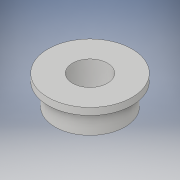
# Autodesk Inventor part: Roller Bearing
Saved by Autodesk Inventor 2019.4 (Build 234330000, 330)
## iProperties
Created: 2020-01-11
Part Number: Roller Bearing
Material: Generic
Document SubType Name: Modeling
Designer: admin
Density: 1 g/cm^3
Appearance: Default
Author: admin
Autodesk Inventor part; units mm, degrees
ref_plane "YZ Plane" through (0, 0, 0) normal (1, 0, 0) x (0, 1, 0)
ref_plane "XZ Plane" through (0, 0, 0) normal (0, 1, 0) x (-1, 0, 0)
ref_plane "XY Plane" through (0, 0, 0) normal (0, 0, 1) x (1, 0, 0)
sketch "Sketch1" plane through (0, 0, 0) normal (1, 0, 0) x (0, 1, 0)
  line L0 (0, 1.5) -> (2.5, 1.5)
  line L1 (2.5, 1.5) -> (2.5, 3.6)
  line L2 (2.5, 3.6) -> (1.9, 3.6)
  line L3 (1.9, 3.6) -> (1.9, 3)
  line L4 (1.9, 3) -> (0, 3)
  line L5 (0, 3) -> (0, 1.5)
  line L6 (-0.5, 0) -> (3, 0) projected
  point P0 (0, 0)
  dimension "d0" = 3
  dimension "d1" = 1.5
  dimension "d2" = 2.5
  dimension "d3" = 0.6
  dimension "d4" = 3.6
  constraints: 12 end point, 5 perpendicular, 1 horizontal, 1 point on line
  measures "d0" distance from line of point (0, 0) L4
  measures "d1" distance from line of point (0, 0) L0
  measures "d2" distance of L0.start L0.end
  measures "d3" distance of L1.end L2.end
  measures "d4" distance from line of point (0, 0) L2
revolve "Revolution1" add sketch "Sketch1" angle 360 about axis through (0, -10, 0) along (0, 1, 0)
body "Solid1"
